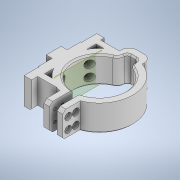
# Autodesk Inventor part: ROOT_CNC_spindel_BTM
Saved by Autodesk Inventor 2020 (Build 240168000, 168)
## iProperties
Created: 2020-07-31
Part Number: ROOT_CNC_spindel_BTM
Material: Générique
Document SubType Name: Modeling
Designer: LounkY
Density: 1 g/cm^3
Appearance: Par défaut
Author: LounkY
Autodesk Inventor part; units mm, degrees
ref_plane "YZ Plane" through (0, 0, 0) normal (1, 0, 0) x (0, 1, 0)
ref_plane "XZ Plane" through (0, 0, 0) normal (0, 1, 0) x (-1, 0, 0)
ref_plane "XY Plane" through (0, 0, 0) normal (0, 0, 1) x (1, 0, 0)
sketch "Esquisse1" plane through (0, 0, 0) normal (0, 1, 0) x (-1, 0, 0)
  circle A0 centre (3.4665, 6.2396) radius 44.2
  point P0 (0, 0)
  dimension "d0" = 88.4
  constraints: 1 centre point
  measures "d0" diameter of A0
extrude "Extrusion1" add sketch "Esquisse1" along normal blind 35
sketch "Esquisse2" plane through (-3.4665, 35, 6.2396) normal (0, 1, 0) x (1, 0, 0)
  circle A0 centre (0, 0) radius 34.25
  circle A1 centre (0, 0) radius 44.2 projected
  point P0 (3.4665, 6.2396)
  dimension "d3" = 68.5
  constraints: 1 centre point, 1 concentric
  measures "d3" diameter of A0
extrude "Extrusion2" cut sketch "Esquisse2" against normal through all contours A0
sketch "Esquisse3" plane through (-3.4665, 35, 6.2396) normal (0, 1, 0) x (1, 0, 0)
  line L0 (-15, 34.25) -> (15, 34.25)
  line L1 (15, 34.25) -> (15, 54.25)
  line L2 (15, 54.25) -> (-15, 54.25)
  line L3 (-15, 54.25) -> (-15, 34.25)
  circle A0 centre (0, 0) radius 34.25 projected
  circle A1 centre (0, 0) radius 44.2 projected
  circle A2 centre (0, 0) radius 34.25 projected
  point P0 (3.4665, 6.2396)
  point P1 (-15, 41.5769)
  point P2 (15, 41.5769)
  dimension "d6" = 20
  dimension "d7" = 30
  dimension "d8" = 15
  dimension "d9" = 9.95
  constraints: 8 end point, 2 parallel, 1 horizontal, 1 perpendicular, 1 tangent
  measures "d6" distance of L0.end L1.end
  measures "d7" distance of L1.end L2.end
  measures "d8" distance from line of A0.centre L3
  measures "d9" radial gap between concentric circles of A1 A0
extrude "Extrusion3" add sketch "Esquisse3" against normal up to surface (35 mm away) contours L3 L2 L1 A1
sketch "Esquisse4" plane through (0, 35, 0) normal (0, 1, 0) x (1, 0, 0)
  line L0 (-10.9665, 23.0104) -> (4.0335, 23.0104)
  line L1 (4.0335, 23.0104) -> (4.0335, 38.0104)
  line L2 (4.0335, 38.0104) -> (-10.9665, 38.0104)
  line L3 (-10.9665, 38.0104) -> (-10.9665, 23.0104)
  line L4 (-18.4665, 48.0104) -> (-18.4665, 35.3373) projected
  line L5 (11.5335, 48.0104) -> (-18.4665, 48.0104) projected
  point P0 (0, 0)
  dimension "d12" = 15
  dimension "d13" = 15
  dimension "d14" = 7.5
  dimension "d15" = 10
  constraints: 8 end point, 2 parallel, 1 horizontal, 1 perpendicular
  measures "d12" distance of L0.end L1.end
  measures "d13" distance of L1.end L2.end
  measures "d14" distance between parallel lines of L3 L4
  measures "d15" distance between parallel lines of L5 L2
extrude "Extrusion4" cut sketch "Esquisse4" against normal up to next
fillet "Congé1" radius 10 4 edges at (-10.9665, 17.5, -27.1791) (4.0335, 17.5, -27.1791) (11.5335, 17.5, -48.0104) (-18.4665, 17.5, -48.0104)
fillet "Congé2" radius 4 2 edges at (-10.9665, 17.5, -38.0104) (4.0335, 17.5, -38.0104)
sketch "Esquisse5" plane through (0, 35, 0) normal (0, 1, 0) x (1, 0, 0)
  line L0 (-12.5, -70.4896) -> (12.5, -70.4896)
  line L1 (12.5, -70.4896) -> (12.5, -40.4896)
  line L2 (12.5, -40.4896) -> (-12.5, -40.4896)
  line L3 (-12.5, -40.4896) -> (-12.5, -70.4896)
  arc A0 (-17.0117, 25.2181) -> (10.0787, 25.2181) centre (-3.4665, -6.2396) ccw projected
  point P0 (0, 0)
  dimension "d20" = 30
  dimension "d21" = 25
  dimension "d22" = 12.5
  constraints: 8 end point, 2 parallel, 1 horizontal, 1 perpendicular, 1 tangent
  measures "d20" distance of L0.end L1.end
  measures "d21" distance of L0.start L0.end
  measures "d22" distance from line of point (0, 0) L1
extrude "Extrusion5" add sketch "Esquisse5" against normal up to surface (35 mm away)
sketch "Esquisse6" plane through (0, 35, 0) normal (0, 1, 0) x (1, 0, 0)
  line L0 (-5, -38.4896) -> (5, -38.4896)
  line L1 (5, -38.4896) -> (5, -70.4896)
  line L2 (5, -70.4896) -> (-5, -70.4896)
  line L3 (-5, -70.4896) -> (-5, -38.4896)
  line L4 (-12.5, -70.4896) -> (12.5, -70.4896) projected
  line L5 (12.5, -70.4896) -> (12.5, -47.4551) projected
  line L6 (-12.5, -49.5066) -> (-12.5, -70.4896) projected
  point P0 (0, 0)
  dimension "d25" = 10
  dimension "d26" = 10
  dimension "d27" = 32
  dimension "d28" = 7.5
  dimension "d29" = 7.5
  constraints: 8 end point, 2 parallel, 1 collinear, 1 horizontal, 1 perpendicular
  measures "d25" distance of L1.end L2.end
  measures "d26" distance of L0.start L0.end
  measures "d27" distance of L0.end L1.end
  measures "d28" distance between parallel lines of L5 L1
  measures "d29" distance between parallel lines of L6 L3
extrude "Extrusion6" cut sketch "Esquisse6" against normal through all
sketch "Esquisse7" plane through (12.5, 35, 70.4896) normal (1, 0, 0) x (0, 0, -1)
  circle A0 centre (7, -10) radius 2
  line L0 (0, 0) -> (0, -35) projected
  line L1 (0, 0) -> (23.0346, 0) projected
  circle A1 centre (17, -10) radius 2
  circle A2 centre (7, -25) radius 2
  circle A3 centre (17, -25) radius 2
  point P0 (70.4896, -35)
  dimension "d32" = 4
  dimension "d33" = 7
  dimension "d34" = 10
  dimension "d37" = 10
  dimension "d40" = 15
  constraints: 4 centre point, 1 horizontal, 1 vertical, 6 other
  measures "d32" diameter of A0
  measures "d33" distance from line of L0 A0.centre
  measures "d34" distance from line of A0.centre L1
  measures "d37" distance of A0.centre A1.centre
  measures "d40" distance of A0.centre A2.centre
extrude "Extrusion7" cut sketch "Esquisse7" against normal up to surface (25 mm away)
chamfer "Chanfrein1" distance 4 angle 45 4 edges at (-8.75, 0, 70.4896) (8.75, 35, 70.4896) (-8.75, 35, 70.4896) (8.75, 0, 70.4896)
sketch "Esquisse10" plane through (0, 35, 0) normal (0, 1, 0) x (1, 0, 0)
  line L0 (-18.4665, 35.3373) -> (-48.4665, 35.3373)
  line L1 (-48.4665, 35.3373) -> (-48.4665, -47.7679)
  line L2 (-48.4665, -47.7679) -> (-18.4665, -47.7679)
  line L3 (-18.4665, -47.7679) -> (-18.4665, 35.3373)
  point P0 (0, 0)
  dimension "d51" = 30
  constraints: 8 end point, 2 parallel, 1 horizontal, 1 perpendicular
  measures "d51" distance of L1.end L2.end
extrude "Extrusion8" add sketch "Esquisse10" against normal up to surface (35 mm away)
sketch "Esquisse11" plane through (0, 35, 0) normal (0, 1, 0) x (1, 0, 0)
  circle A0 centre (-3.4665, -6.2396) radius 34.25
  arc A1 (5, -39.4267) -> (10.0787, 25.2181) centre (-3.4665, -6.2396) ccw projected
  point P0 (0, 0)
  dimension "d54" = 68.5
  constraints: 1 centre point, 1 concentric
  measures "d54" diameter of A0
extrude "Extrusion9" cut sketch "Esquisse11" against normal through all
sketch "Esquisse12" plane through (0, 35, 0) normal (0, 1, 0) x (1, 0, 0)
  circle A0 centre (-3.4665, -6.2396) radius 44.2
  arc A1 (12.5, -47.4551) -> (11.5335, 35.3373) centre (-3.4665, -6.2396) ccw projected
  line L0 (-41.9551, 27.8373) -> (-31.6161, 27.8373)
  line L1 (-31.6751, -40.2677) -> (-41.9551, -40.2677)
  line L2 (-18.4665, 35.3373) -> (-48.4665, 35.3373) projected
  line L3 (-41.9551, -40.2677) -> (-41.9551, -27.9713)
  line L4 (-41.9551, 15.4921) -> (-41.9551, 27.8373)
  point P0 (0, 0)
  dimension "d57" = 88.4
  dimension "d58" = 68.105
  dimension "d59" = 7.5
  constraints: 8 end point, 4 point on circle, 1 centre point, 1 concentric, 1 horizontal, 1 parallel
  measures "d57" diameter of A0
  measures "d58" distance of L1.end L0.start
  measures "d59" distance between parallel lines of L0 L2
extrude "Extrusion10" cut sketch "Esquisse12" against normal through all contours L1 L3 A0 | A0 L4 L0
sketch "Esquisse13" plane through (-48.4665, 35, -35.3373) normal (-1, 0, 0) x (0, 0, 1)
  line L0 (-4.9475, 0) -> (91.0525, 0)
  line L1 (91.0525, 0) -> (91.0525, -35)
  line L2 (91.0525, -35) -> (-4.9475, -35)
  line L3 (-4.9475, -35) -> (-4.9475, 0)
  line L4 (0, 0) -> (83.1052, 0) projected
  line L5 (0, 0) -> (0, -35) projected
  point P0 (35.3373, -35)
  dimension "d62" = 96
  dimension "d63" = 35
  dimension "d64" = 4.9475
  dimension "d65" = 83.1052
  dimension "d66" = 96
  constraints: 8 end point, 2 parallel, 1 collinear, 1 horizontal, 1 perpendicular
  measures "d62" distance of L0.start L0.end
  measures "d63" distance of L2.end L0.start
  measures "d64" distance between parallel lines of L5 L3
  measures "d65" distance of L4.end L4.start
  measures "d66" distance of L1.end L2.end
extrude "Extrusion11" add sketch "Esquisse13" along normal mid plane 10
sketch "Esquisse14" plane through (-53.4665, 35, -35.3373) normal (-1, 0, 0) x (0, 0, 1)
  line L0 (75.7926, -35) -> (10.1192, -35) projected
  line L1 (15.0525, 0) -> (71.0525, 0)
  line L2 (71.0525, 0) -> (71.0525, -35)
  line L3 (71.0525, -35) -> (15.0525, -35)
  line L4 (15.0525, -35) -> (15.0525, 0)
  line L5 (91.0525, -35) -> (91.0525, 0) projected
  point P0 (35.3373, -35)
  point P1 (15.0525, -35)
  dimension "d69" = 56
  dimension "d70" = 20
  constraints: 8 end point, 2 parallel, 1 horizontal, 1 perpendicular, 1 point on line
  measures "d69" distance of L1.start L1.end
  measures "d70" distance between parallel lines of L5 L2
extrude "Extrusion12" add sketch "Esquisse14" along normal mid plane 2
sketch "Esquisse15" plane through (-54.4665, 35, -35.3373) normal (-1, 0, 0) x (0, 0, 1)
  line L0 (10.1192, 0) -> (74.764, 0) projected
  line L1 (33.1525, 0) -> (52.9525, 0)
  line L2 (52.9525, 0) -> (52.9525, -12.8)
  line L3 (52.9525, -12.8) -> (33.1525, -12.8)
  line L4 (33.1525, -12.8) -> (33.1525, 0)
  line L5 (15.0525, 0) -> (15.0525, -35) projected
  line L6 (74.764, -35) -> (10.1192, -35) projected
  line L7 (52.9525, -35) -> (33.1525, -35)
  line L8 (33.1525, -35) -> (33.1525, -22.2)
  line L9 (33.1525, -22.2) -> (52.9525, -22.2)
  line L10 (52.9525, -22.2) -> (52.9525, -35)
  point P0 (35.3373, -35)
  dimension "d73" = 19.8
  dimension "d74" = 18.1
  dimension "d75" = 12.8
  dimension "d76" = 12.8
  constraints: 16 end point, 4 parallel, 2 horizontal, 2 perpendicular, 2 point on line
  measures "d73" distance of L2.end L3.end
  measures "d74" distance between parallel lines of L5 L4
  measures "d75" distance of L1.end L2.end
  measures "d76" distance of L9.end L7.start
extrude "Extrusion13" add sketch "Esquisse15" along normal blind 8
sketch "Esquisse16" plane through (-54.4665, 35, -35.3373) normal (-1, 0, 0) x (0, 0, 1)
  circle A0 centre (25.0525, -10) radius 3
  line L0 (33.1525, 0) -> (33.1525, -12.8) projected
  line L1 (33.1525, 0) -> (15.0525, 0) projected
  circle A1 centre (61.0525, -10) radius 3
  line L2 (15.0525, 0) -> (15.0525, -35) projected
  circle A2 centre (25.0525, -25) radius 3
  circle A3 centre (61.0525, -25) radius 3
  point P0 (35.3373, -35)
  dimension "d79" = 6
  dimension "d80" = 8.1
  dimension "d81" = 10
  dimension "d84" = 36
  dimension "d89" = 10
  dimension "d92" = 15
  dimension "d97" = 6
  dimension "d98" = 15
  dimension "d99" = 36
  constraints: 4 centre point, 1 horizontal, 1 vertical, 4 other
  measures "d79" diameter of A0
  measures "d80" distance from line of A0.centre L0
  measures "d81" distance from line of A0.centre L1
  measures "d84" distance of A0.centre A1.centre
  measures "d89" distance from line of L2 A0.centre
  measures "d92" distance of A0.centre A2.centre
  measures "d97" diameter of A3
  measures "d98" distance of A3.centre A1.centre
  measures "d99" distance of A3.centre A2.centre
extrude "Extrusion14" cut sketch "Esquisse16" against normal up to surface
ref_plane "Plan de construction2" through (-29.9665, 35, -35.3373) normal (-1, 0, 0) x (0, 0, 1)
sketch "Esquisse19" plane through (-29.9665, 35, -35.3373) normal (-1, 0, 0) x (0, 0, 1)
  circle A0 centre (25.0525, -25) radius 3 projected
  circle A1 centre (25.0525, -25) radius 5
  circle A2 centre (61.0525, -25) radius 3 projected
  circle A3 centre (61.0525, -25) radius 5
  circle A4 centre (61.0525, -10) radius 3 projected
  circle A5 centre (61.0525, -10) radius 5
  circle A6 centre (25.0525, -10) radius 3 projected
  circle A7 centre (25.0525, -10) radius 5
  point P0 (35.3373, -35)
  dimension "d104" = 10
  dimension "d105" = 10
  dimension "d106" = 10
  dimension "d107" = 10
  constraints: 4 centre point, 4 coincident
  measures "d104" diameter of A1
  measures "d105" diameter of A5
  measures "d106" diameter of A7
  measures "d107" diameter of A3
extrude "Extrusion15" cut sketch "Esquisse19" along normal blind 8 contours A0 | A1 | A2 | A3 | A4 | A5 | A6 | A7
sketch "Esquisse20" plane through (12.5, 4, 70.4896) normal (1, 0, 0) x (0, 0, -1)
  circle A0 centre (7, 21) radius 2 projected
  circle A1 centre (7, 21) radius 4.5
  circle A2 centre (17, 21) radius 2 projected
  circle A3 centre (17, 21) radius 4.5
  circle A4 centre (17, 6) radius 4.5
  circle A5 centre (7, 6) radius 4.5
  circle A6 centre (7, 21) radius 2 projected
  circle A7 centre (17, 6) radius 2 projected
  circle A8 centre (7, 6) radius 2 projected
  point P0 (70.4896, -4)
  dimension "d113" = 9
  dimension "d114" = 9
  dimension "d115" = 9
  dimension "d116" = 9
  constraints: 4 centre point, 3 concentric, 2 coincident
  measures "d113" diameter of A1
  measures "d114" diameter of A3
  measures "d115" diameter of A4
  measures "d116" diameter of A5
extrude "Extrusion16" cut sketch "Esquisse20" against normal blind 4
chamfer "Chanfrein3" distance 2 angle 45 33 edges at (30.6783, 0, 8.9222) (5.7584, 0, -28.7885) (2.8275, 0, -36.8782) (-3.4665, 0, -38.0104) (-9.7605, 0, -36.8782) (-12.6913, 0, -28.7885) (-37.1576, 0, 12.4017) (40.7305, 0, 5.7237) (12.5, 0, 56.9723) (-12.5, 0, 57.9981) (-31.0335, 0, 47.7679) (-43.4665, 0, -37.811) (-43.4665, 0, 51.7416) (-30.9665, 0, -35.3373) (-3.4665, 0, -48.0104) (8.6046, 0, -45.0814) (11.5335, 0, -36.6738) (-15.5375, 0, -45.0814) (-18.4665, 0, -36.6738) (-15.5815, 0, 48.7469) (-37.3771, 0, 34.5894) (-36.8151, 0, 40.2677) (-41.9551, 0, 34.1195) (-41.9551, 0, -21.6647) (-37.3525, 0, -22.1395) (-36.7856, 0, -27.8373) (-37.1576, 35, 12.4017) (-12.6913, 35, -28.7885) (-9.7605, 35, -36.8782) (-3.4665, 35, -38.0104) (2.8275, 35, -36.8782) (5.7584, 35, -28.7885) (30.6783, 35, 8.9222)
